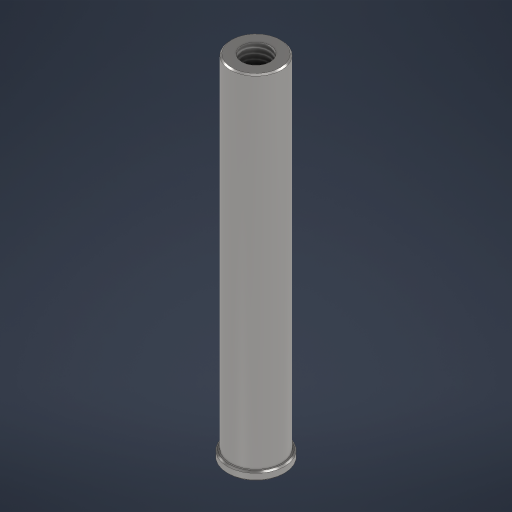
# Autodesk Inventor part: Z25_Hinge_Shaft
Saved by Autodesk Inventor 2024.1 (Build 281209000, 209)
## iProperties
Created: 2023-02-13
Part Number: Z25_Hinge_Shaft
Material: Stainless Steel
Document SubType Name: Modeling
Designer: dzw04
Density: 8 g/cm^3
Appearance: Semi-Polished
Author: dzw04
Autodesk Inventor part; units mm, degrees
ref_plane "YZ Plane" through (0, 0, 0) normal (1, 0, 0) x (0, 1, 0)
ref_plane "XZ Plane" through (0, 0, 0) normal (0, 1, 0) x (-1, 0, 0)
ref_plane "XY Plane" through (0, 0, 0) normal (0, 0, 1) x (1, 0, 0)
sketch "Sketch1" plane through (0, 0, 0) normal (0, 1, 0) x (-1, 0, 0)
  circle A0 centre (0, 0) radius 2.5
  dimension "d0" = 5
  constraints: 1 centre point, 1 coincident
  measures "d0" diameter of A0
extrude "Extrusion1" add sketch "Sketch1" along normal blind 0.75
chamfer "Chamfer1" distance 0.125 angle 45 2 edges at (2.5, 0, 0) (2.5, 0.75, 0)
sketch "Sketch2" plane through (0, 0.75, 0) normal (0, 1, 0) x (1, 0, 0)
  circle A0 centre (0, 0) radius 2.25
  dimension "d6" = 4.5
  constraints: 1 centre point, 1 coincident
  measures "d6" diameter of A0
extrude "Extrusion2" add sketch "Sketch2" along normal blind 30
sketch "Sketch3" plane through (0, 30.75, 0) normal (0, 1, 0) x (1, 0, 0)
  circle A0 centre (0, 0) radius 1.25
  dimension "d9" = 2.5
  constraints: 1 centre point, 1 coincident
  measures "d9" diameter of A0
extrude "Extrusion3" cut sketch "Sketch3" against normal blind 5
thread "Thread1" size "M2.5x0.45" class "6H" standard "ANSI Metric M Profile" full length
chamfer "Chamfer2" distance 0.125 angle 45 1 edges at (-2.25, 30.75, 0)
body "Solid1"
